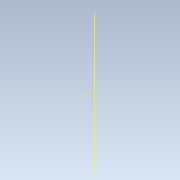
# Autodesk Inventor part: cinta_protectora
Saved by Autodesk Inventor 2021 (Build 250183000, 183)
## iProperties
Created: 2021-04-15
Part Number: cinta_protectora
Material: Genérico
Document SubType Name: Modeling
Designer: j2seb
Density: 1 g/cm^3
Appearance: Valor por defecto
Author: j2seb
Autodesk Inventor part; units mm, degrees
ref_plane "YZ Plane" through (0, 0, 0) normal (1, 0, 0) x (0, 1, 0)
ref_plane "XZ Plane" through (0, 0, 0) normal (0, 1, 0) x (-1, 0, 0)
ref_plane "XY Plane" through (0, 0, 0) normal (0, 0, 1) x (1, 0, 0)
sketch "Boceto2" plane through (0, 0, 0) normal (0, 0, 1) x (1, 0, 0)
  spline S0 degree 5 poles (-24.9404, 274.1789) (-19.9523, 272.5074) (-14.9642, 271.2537) (-9.9761, 270.4179) (0, 269.5821) (9.9761, 270.4179) (14.9642, 271.2537) (19.9523, 272.5074) (24.9404, 274.1789) knots 0 0 0 0 0 0 25.288037 25.288037 25.288037 50.576075 50.576075 50.576075 50.576075 50.576075 50.576075 projected
  line L0 (-20, 272.6873) -> (-20, 273.7233)
  line L1 (20, 272.6873) -> (20, 273.7233)
  line L2 (0, 271) -> (0, 0) construction
  line L3 (-60, 0) -> (55, 0)
  spline S1 degree 5 poles (-20, 273.7233) (-16.0933, 272.6596) (-12.1209, 271.8375) (-8.0978, 271.279) (0, 270.721) (8.0978, 271.279) (12.1209, 271.8375) (16.0933, 272.6596) (20, 273.7233) knots 0 0 0 0 0 0 0.5 0.5 0.5 1 1 1 1 1 1
  dimension "d0" = 1
  dimension "d1" = 20
  dimension "d2" = 20
  constraints: 8 end point, 3 vertical, 1 horizontal, 1 point on line, 6 other
  measures "d1" distance between parallel lines of L0 L2
  measures "d2" distance between parallel lines of L1 L2
revolve "Revolución1" add sketch "Boceto2" angle 360 about axis through (-60, 0, 0) along (1, 0, 0)
